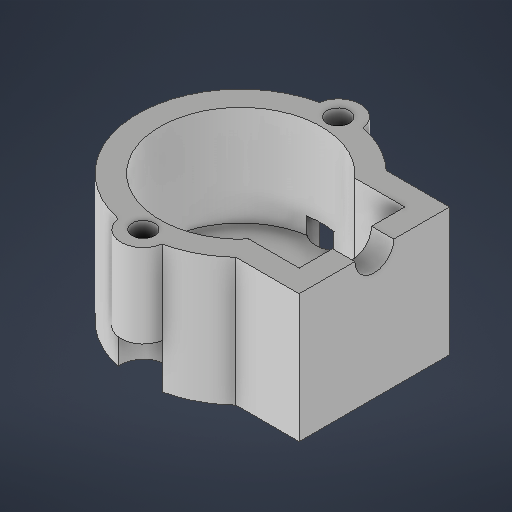
# Autodesk Inventor part: motor_holder_v2
Saved by Autodesk Inventor 2026.2 (Build 302298000, 298)
## iProperties
Created: 2026-01-14
Part Number: motor_holder_v2
Material: Generic
Document SubType Name: Modeling
Designer: User
Density: 1 g/cm^3
Appearance: Default
Author: User
Autodesk Inventor part; units mm, degrees
ref_plane "YZ Plane" through (0, 0, 0) normal (1, 0, 0) x (0, 1, 0)
ref_plane "XZ Plane" through (0, 0, 0) normal (0, 1, 0) x (-1, 0, 0)
ref_plane "XY Plane" through (0, 0, 0) normal (0, 0, 1) x (1, 0, 0)
sketch "Sketch1" plane through (0, 0, 0) normal (0, 1, 0) x (-1, 0, 0)
  arc A0 (-9.5, 10.9545) -> (9.5, 10.9545) centre (0, 0) ccw
  line L0 (-9.5, 10.9545) -> (-9.5, 20)
  line L1 (-9.5, 20) -> (9.5, 20)
  line L2 (9.5, 20) -> (9.5, 10.9545)
  line L3 (13.5, 12.6491) -> (13.5, 24)
  line L4 (13.5, 24) -> (-13.5, 24)
  line L5 (-13.5, 24) -> (-13.5, 12.6491)
  arc A1 (-13.5, 12.6491) -> (13.5, 12.6491) centre (0, 0) ccw
  point P0 (0, -20)
  point P1 (-9.5, 15)
  dimension "d0" = 0
  dimension "d1" = 29
  dimension "d6" = 20
  dimension "d7" = 19
  dimension "d8" = 4
  constraints: 12 end point, 4 point on circle, 2 centre point, 2 parallel, 1 coincident, 1 point on line, 3 other
  measures "d0" horizontal distance of A0.centre point (0, -20)
  measures "d1" diameter of A0
  measures "d6" distance from line of L1 point (0, 0)
  measures "d7" distance of L0.end L1.end
  measures "d8" radial gap between concentric circles of A0 A1
extrude "Extrusion1" add sketch "Sketch1" along normal blind 18
sketch "Sketch2" plane through (0, 18, 0) normal (0, 1, 0) x (1, 0, 0)
  arc A0 (13.5, -12.6491) -> (-13.5, -12.6491) centre (0, 0) ccw
  line L0 (-13.5, -12.6491) -> (-13.5, -24) projected
  line L1 (-13.5, -24) -> (13.5, -24)
  line L2 (13.5, -24) -> (13.5, -12.6491)
  line L3 (-13.5, -12.6491) -> (-13.5, -24)
  constraints: 6 end point, 2 point on circle, 1 centre point, 1 coincident, 1 horizontal, 1 parallel, 1 perpendicular
extrude "Extrusion2" add sketch "Sketch2" along normal blind 5
sketch "Sketch3" plane through (-13.5, 0, 24) normal (0, 0, 1) x (1, 0, 0)
  circle A0 centre (13.5, 0) radius 3.5
  dimension "d13" = 7
  constraints: 1 centre point, 1 coincident
  measures "d13" diameter of A0
extrude "Extrusion3" cut sketch "Sketch3" against normal blind 5
sketch "Sketch7" plane through (0, 0, 0) normal (0, -1, 0) x (1, 0, 0)
  circle A0 centre (-17.5, 0) radius 2
  circle A1 centre (17.5, 0) radius 2
  arc A2 (-18.0714, 3.959) -> (-18.0714, -3.959) centre (-17.5, 0) ccw
  arc A3 (18.0714, -3.959) -> (18.0714, 3.959) centre (17.5, 0) ccw
  arc A4 (-13.5, 12.6491) -> (13.5, 12.6491) centre (0, 0) ccw projected
  point P0 (18.4143, 1.7788)
  point P1 (18.4143, -1.7788)
  point P2 (-18.4143, -1.7788)
  point P3 (-18.4143, 1.7788)
  dimension "d29" = 4
  dimension "d30" = 4
  dimension "d31" = 35
  dimension "d32" = 17.5
  dimension "d33" = 8
  dimension "d34" = 8
  constraints: 8 point on circle, 4 centre point, 2 coincident, 2 horizontal alignment
  measures "d29" diameter of A0
  measures "d30" diameter of A1
  measures "d31" distance of A1.centre A0.centre
  measures "d32" distance of point (0, 0) A0.centre
  measures "d33" diameter of A2
  measures "d34" diameter of A3
extrude "Extrusion6" add sketch "Sketch7" against normal blind 15 contours A0 A4 A2 | A1 A4 A3
extrude "Extrusion7" cut sketch "Sketch7" against normal blind 15 contours A0 A4 | A4 A1 picked at (-17.4936, 0) picked at (17.4985, 0.08)
sketch "Sketch8" plane through (0, 0, 0) normal (0, 0, 1) x (1, 0, 0)
  line L0 (17.5, 15) -> (21.5, 15)
  line L1 (21.5, 15) -> (21.5, 19)
  line L2 (21.5, 19) -> (17.5, 19)
  line L3 (17.5, 19) -> (17.5, 15)
  line L4 (18.0714, 0) -> (-18.0714, 0) projected
  line L5 (21.5, 15) -> (18.0714, 15) projected
  point P0 (0, 0)
  point P1 (0, 0)
  dimension "d39" = 17.5
  dimension "d40" = 0
  dimension "d41" = 4
  dimension "d42" = 4
  constraints: 8 end point, 2 parallel, 1 horizontal, 1 midpoint, 1 perpendicular
  measures "d39" distance from line of point (0, 0) L3
  measures "d40" distance between parallel lines of L5 L0
  measures "d41" distance of L1.end L2.end
  measures "d42" distance of L0.end L1.end
revolve "Revolution1" cut sketch "Sketch8" angle 360 about axis through (17.5, 19, 0) along (0, -1, 0)
sketch "Sketch9" plane through (17.5, 19, 0) normal (0, -1, 0) x (1, 0, 0)
  arc A0 (0.5714, 3.959) -> (0.5714, -3.959) centre (0, 0) ccw projected
  point P0 (-17.5, 0)
  constraints: 1 coincident
hole "Hole1" at (17.5, 19, 0) direction (0, 1, 0) diameter 8 end through all
mirror "Mirror1" about plane through (0, 0, 0) normal (1, 0, 0) of "Revolution1"
sketch "Sketch10" plane through (-17.5, 19, 0) normal (0, -1, 0) x (1, 0, 0)
  arc A0 (3.2, -2.4) -> (3.2, 2.4) centre (0, 0) ccw projected
  point P0 (17.5, 0)
  constraints: 1 coincident
hole "Hole2" at (-17.5, 19, 0) direction (0, 1, 0) diameter 8 end through all
body "Solid1"
